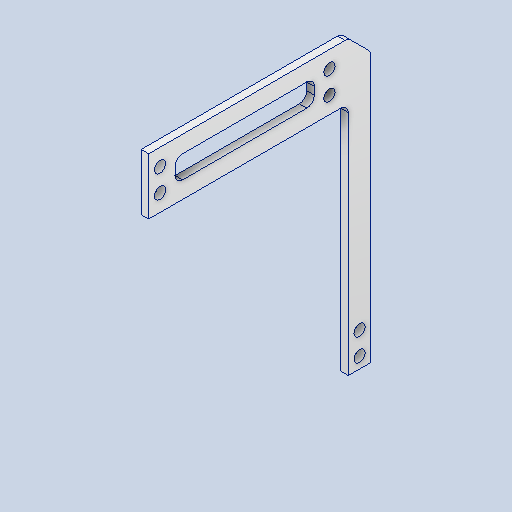
# Autodesk Inventor part: Plate_Support
Saved by Autodesk Inventor 2025.3 (Build 293356000, 356)
## iProperties
Created: 2026-08-26
Part Number: Plate_Support
Material: アルミニウム 6061
Document SubType Name: Modeling
Designer: tanan
Density: 2.7 g/cm^3
Appearance: アルミニウム - フラット
Author: tanan
Autodesk Inventor part; units mm, degrees
ref_plane "YZ Plane" through (0, 0, 0) normal (1, 0, 0) x (0, 1, 0)
ref_plane "XZ Plane" through (0, 0, 0) normal (0, 1, 0) x (-1, 0, 0)
ref_plane "XY Plane" through (0, 0, 0) normal (0, 0, 1) x (1, 0, 0)
sketch "スケッチ1" plane through (0, 0, 0) normal (1, 0, 0) x (0, 1, 0)
  line L0 (0, 0) -> (15, 0)
  line L1 (15, 0) -> (15, -53)
  line L2 (15, -53) -> (0, -53)
  line L3 (0, -53) -> (0, 0)
  line L4 (9, -53) -> (-62.5, -53)
  line L5 (-62.5, -53) -> (-62.5, -59)
  line L6 (-62.5, -59) -> (9, -59)
  line L7 (9, -59) -> (9, -53)
  line L8 (15, -53) -> (9, -59)
  line L9 (0, -53) -> (0, -53)
  line L10 (10.5, -3) -> (4.5, -3)
  line L11 (4.5, -3) -> (4.5, -48)
  line L12 (4.5, -48) -> (10.5, -48)
  line L13 (10.5, -48) -> (10.5, -3)
  line L14 (15, -50.5) -> (0, -50.5)
  point P0 (7.5, 0)
  point P1 (7.5, -3)
  point P2 (-53.5, -56)
  point P3 (-59.5, -56)
  point P4 (-62.5, -56)
  dimension "d0" = 53
  dimension "d4" = 6
  dimension "d5" = 3
  dimension "d6" = 5
  dimension "d22" = 4.5
  dimension "d23" = 6
  dimension "d24" = 6
  dimension "d25" = 3
  dimension "d26" = 73
  dimension "d27" = 2.5
  dimension "d28" = 2.5
  dimension "d29" = 135
  constraints: 30 end point, 6 parallel, 4 horizontal, 4 perpendicular, 3 midpoint, 3 point on line, 2 horizontal alignment, 1 vertical alignment
  measures "d0" distance between parallel lines of L0 L2
  measures "d4" distance of L10.start L10.end
  measures "d5" distance from line of point (7.5, 0) L10
  measures "d6" distance between parallel lines of L2 L12
  measures "d22" distance between parallel lines of L3 L11
  measures "d23" distance of L4.end L5.end
  measures "d24" distance of point (-59.5, -56) point (-53.5, -56)
  measures "d25" distance from line of L5 point (-59.5, -56)
  measures "d26" distance between parallel lines of L5 L13
  measures "d27" distance between parallel lines of L12 L14
  measures "d28" distance between parallel lines of L14 L4
  measures "d29" angle of L1 L8
extrude "押し出し1" add sketch "スケッチ1" along normal blind 2 contours L0 L1 L14 L3 | L14 L1 L2 L3 | L2 L7 L6 L5 L4 | L8 L7 L2 | L13 L12 L11 L10
hole "穴1" at (0, 10.5, -3) at (0, 4.5, -3) at (0, 10.5, -48) at (0, 4.5, -48) at (0, -53.5, -56) at (0, -59.5, -56) direction (1, 0, 0) diameter 3 depth 8.8
sketch "スケッチ2" plane through (2, 0, 0) normal (1, 0, 0) x (0, 0, -1)
  line L0 (9, 10.5) -> (42, 10.5)
  line L1 (44, 8.5) -> (44, 6.5)
  line L2 (42, 4.5) -> (9, 4.5)
  line L3 (7, 6.5) -> (7, 8.5)
  line L4 (0, 15) -> (0, 0) projected
  circle A0 centre (3, 10.5) radius 1.5 projected
  circle A1 centre (48, 10.5) radius 1.5 projected
  arc A2 (9, 10.5) -> (7, 8.5) centre (9, 8.5) ccw
  arc A3 (7, 6.5) -> (9, 4.5) centre (9, 6.5) ccw
  arc A4 (42, 4.5) -> (44, 6.5) centre (42, 6.5) ccw
  arc A5 (44, 8.5) -> (42, 10.5) centre (42, 8.5) ccw
  point P0 (44, 10.5)
  point P1 (7, 7.5)
  point P2 (0, 7.5)
  dimension "d16" = 4
  dimension "d17" = 4
  dimension "d18" = 2
  constraints: 8 end point, 8 point on circle, 8 tangent, 4 centre point, 3 equal radius, 2 horizontal alignment, 2 midpoint, 2 parallel, 2 point on line, 1 horizontal, 1 perpendicular
  measures "d16" distance from line of L3 A0.centre
  measures "d17" distance from line of A1.centre L1
  measures "d18" radius of A2
extrude "押し出し2" cut sketch "スケッチ2" against normal blind 2 contours L0 A5 L1 A4 L2 A3 L3 A2
fillet "フィレット1" radius 2 1 edges at (1, 15, -53)
fillet "フィレット2" radius 2 2 edges at (1, 9, -59) (1, 0, -53)
equation "\"d1\" = 1"
